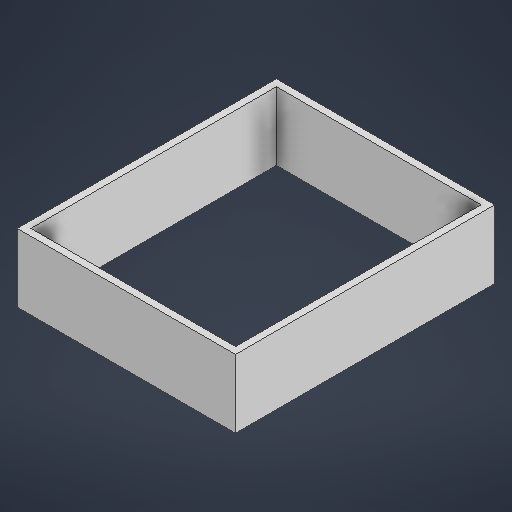
# Autodesk Inventor part: CaseBitDog
Saved by Autodesk Inventor 2027 (Build 310192000, 192)
## iProperties
Created: 2026-10-02
Part Number: CaseBitDog
Material: Genérico
Document SubType Name: Modeling
Designer: EspacoMaker
Density: 1 g/cm^3
Appearance: Padrão
Author: EspacoMaker
Autodesk Inventor part; units mm, degrees
ref_plane "YZ Plane" through (0, 0, 0) normal (1, 0, 0) x (0, 1, 0)
ref_plane "XZ Plane" through (0, 0, 0) normal (0, 1, 0) x (-1, 0, 0)
ref_plane "XY Plane" through (0, 0, 0) normal (0, 0, 1) x (1, 0, 0)
sketch "Esboço1" plane through (0, 0, 0) normal (0, 1, 0) x (-1, 0, 0)
  line L0 (75, 90) -> (-75, 90)
  line L1 (-75, 90) -> (-75, -90)
  line L2 (-75, -90) -> (75, -90)
  line L3 (75, -90) -> (75, 90)
  line L4 (75, 90) -> (-75, -90) construction
  line L5 (-75, 90) -> (75, -90) construction
  line L6 (50.5, 80) -> (-50.5, 80) construction
  line L7 (-50.5, 80) -> (-50.5, -8) construction
  line L8 (-50.5, -8) -> (50.5, -8) construction
  line L9 (50.5, -8) -> (50.5, 80) construction
  line L10 (50.5, 80) -> (-50.5, -8) construction
  line L11 (-50.5, 80) -> (50.5, -8) construction
  line L12 (35, -30) -> (-35, -30) construction
  line L13 (-35, -30) -> (-35, -80) construction
  line L14 (-35, -80) -> (35, -80) construction
  line L15 (35, -80) -> (35, -30) construction
  line L16 (35, -30) -> (-35, -80) construction
  line L17 (-35, -30) -> (35, -80) construction
  line L18 (0, 90) -> (0, -90) construction
  line L19 (80, 95) -> (-80, 95)
  line L20 (-80, 95) -> (-80, -95)
  line L21 (-80, -95) -> (80, -95)
  line L22 (80, -95) -> (80, 95)
  point P0 (0, 0)
  point P1 (0, 36)
  point P2 (0, -55)
  dimension "d0" = 150
  dimension "d1" = 180
  dimension "d2" = 101
  dimension "d3" = 88
  dimension "d4" = 70
  dimension "d5" = 50
  dimension "d6" = 10
  dimension "d7" = 10
  dimension "d8" = 5
  constraints: 46 end point, 8 midpoint, 8 parallel, 4 perpendicular, 3 horizontal, 2 point on line, 3 other
  measures "d0" distance of L2.end L1.end
  measures "d1" distance of L1.end L0.end
  measures "d2" distance of L8.end L7.end
  measures "d3" distance of L7.end L6.end
  measures "d4" distance of L14.end L13.end
  measures "d5" distance of L13.end L12.end
  measures "d6" distance between parallel lines of L2 L14
  measures "d7" distance between parallel lines of L0 L6
  measures "d8" distance between parallel lines of L3 L22
extrude "Extrusão1" add sketch "Esboço1" along normal blind 50
